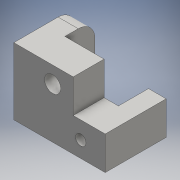
# Autodesk Inventor part: 240503_3Dsketch11
Saved by Autodesk Inventor 2016 (Build 200138000, 138)
## iProperties
Created: 2024-05-03
Part Number: 240503_3Dsketch11
Material: 일반
Document SubType Name: Modeling
Designer: pc
Density: 1 g/cm^3
Appearance: 기본값
Author: pc
Autodesk Inventor part; units mm, degrees
ref_plane "YZ Plane" through (0, 0, 0) normal (1, 0, 0) x (0, 1, 0)
ref_plane "XZ Plane" through (0, 0, 0) normal (0, 1, 0) x (-1, 0, 0)
ref_plane "XY Plane" through (0, 0, 0) normal (0, 0, 1) x (1, 0, 0)
sketch "스케치1" plane through (0, 0, 0) normal (0, 0, 1) x (1, 0, 0)
  line L0 (13.6602, -9.1135) -> (-13.6602, -9.1135)
  line L1 (-13.6602, -9.1135) -> (-13.6602, 9.1135)
  line L2 (-13.6602, 9.1135) -> (13.6602, 9.1135)
  line L3 (13.6602, 9.1135) -> (13.6602, -9.1135)
  line L4 (13.6602, -9.1135) -> (-13.6602, 9.1135) construction
  line L5 (-13.6602, -9.1135) -> (13.6602, 9.1135) construction
  point P0 (0, 0)
  constraints: 12 end point, 2 midpoint, 2 parallel, 1 horizontal, 1 perpendicular
extrude "돌출1" add sketch "스케치1" along normal blind 20
sketch "스케치2" plane through (-13.6602, 9.1135, 0) normal (0, 1, 0) x (1, 0, 0)
  line L0 (0, -20) -> (27.3204, -20) projected
  line L1 (27.3204, 0) -> (27.3204, -20) projected
  line L2 (17.7495, -20) -> (27.3204, -20)
  line L3 (27.3204, -20) -> (27.3204, -10)
  line L4 (27.3204, -10) -> (17.7495, -10)
  line L5 (17.7495, -10) -> (17.7495, -20)
  point P0 (13.6602, 0)
  constraints: 8 end point, 2 parallel, 1 horizontal, 1 midpoint, 1 perpendicular, 1 point on line
extrude "돌출2" cut sketch "스케치2" against normal blind 20
sketch "스케치3" plane through (-13.6602, 9.1135, 0) normal (0, 1, 0) x (1, 0, 0)
  point P0 (13.6602, 0)
sketch "스케치4" plane through (-13.6602, 9.1135, 0) normal (0, 1, 0) x (1, 0, 0)
  line L0 (0, -20) -> (17.7495, -20) projected
  line L1 (6.0281, -20) -> (6.0281, 0)
  line L2 (27.3204, 0) -> (0, 0) projected
  line L3 (22.0453, 0) -> (22.0453, -10)
  line L4 (17.7495, -10) -> (27.3204, -10) projected
  line L5 (17.7495, -20) -> (17.7495, -10) projected
  line L6 (17.7495, -10) -> (17.7495, -20)
  line L7 (17.7495, -20) -> (6.0281, -20)
  point P0 (13.6602, 0)
  constraints: 8 end point, 4 point on line, 2 collinear, 1 parallel, 1 vertical
extrude "돌출3" cut sketch "스케치4" against normal blind 9
sketch "스케치5" plane through (-13.6602, 0.1135, 0) normal (0, 1, 0) x (1, 0, 0)
  circle A0 centre (20.026, -4.8257) radius 1.5639
  circle A1 centre (11.6067, -15.0931) radius 2.4307
  point P0 (13.6602, 0)
  constraints: 2 centre point
extrude "돌출4" cut sketch "스케치5" against normal blind 10
fillet "모깎기1" radius 5 1 edges at (-10.6462, 9.1135, 20)
fillet "모깎기2" radius 5 1 edges at (-10.6462, 9.1135, 0)
